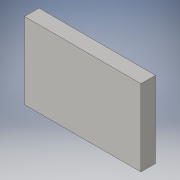
# Autodesk Inventor part: SumoBotCad Pt.1
Saved by Autodesk Inventor 2016 (Build 200138000, 138)
## iProperties
Created: 2017-08-31
Part Number: SumoBotCad Pt.1
Material: Generic
Document SubType Name: Modeling
Designer: Student
Density: 1 g/cm^3
Appearance: Default
Author: Student
Autodesk Inventor part; units mm, degrees
ref_plane "YZ Plane" through (0, 0, 0) normal (1, 0, 0) x (0, 1, 0)
ref_plane "XZ Plane" through (0, 0, 0) normal (0, 1, 0) x (-1, 0, 0)
ref_plane "XY Plane" through (0, 0, 0) normal (0, 0, 1) x (1, 0, 0)
sketch "Sketch3" plane through (0, 0, 0) normal (0, 0, 1) x (1, 0, 0)
  line L0 (40, -26.25) -> (-40, -26.25)
  line L1 (-40, -26.25) -> (-40, 26.25)
  line L2 (-40, 26.25) -> (40, 26.25)
  line L3 (40, 26.25) -> (40, -26.25)
  line L4 (40, -26.25) -> (-40, 26.25) construction
  line L5 (-40, -26.25) -> (40, 26.25) construction
  point P0 (0, 0)
  dimension "d8" = 80
  dimension "d9" = 52.5
  constraints: 12 end point, 2 midpoint, 2 parallel, 1 horizontal, 1 perpendicular
  measures "d8" distance of L1.end L2.end
  measures "d9" distance of L0.end L1.end
extrude "Extrusion2" add sketch "Sketch3" along normal blind 10
body "Solid2"
